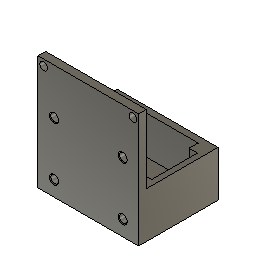
DigitalRegulator_mount_base v4 (Autodesk Fusion 360 design; units mm, degrees)
Autodesk Fusion 360 part; units mm, degrees
sketch "Sketch1" plane through (0, 0, 0) normal (0, 0, 1) x (1, 0, 0)
  line L0 (0, 0) -> (60, 0)
  line L1 (60, 0) -> (60, 50)
  line L2 (60, 50) -> (0, 50)
  line L3 (0, 50) -> (0, 0)
  dimension "d1" = 60
  dimension "d2" = 50
  constraint horizontal L0
  constraint vertical L1
  constraint horizontal L2
  constraint vertical L3
  constraint coincident L0.start L3.end
  measures "d1" distance of L0.start L0.end
  measures "d2" distance of L0.start L2.end
extrude "Extrude1" add sketch "Sketch1" along normal blind 30
sketch "Sketch2" plane through (0, 0, 30) normal (0, 0, 1) x (-1, 0, 0)
  line L0 (0, -50) -> (0, 0)
  line L1 (0, 0) -> (-60, 0)
  line L2 (-60, 0) -> (-60, -50)
  line L3 (-60, -50) -> (0, -50)
  line L4 (-54, -5) -> (-6, -5)
  line L5 (-6, -5) -> (-6, -45)
  line L6 (-6, -45) -> (-54, -45)
  line L7 (-54, -45) -> (-54, -5)
  line L8 (-54, -5) -> (-6, -45) construction
  line L9 (-6, -5) -> (-54, -45) construction
  point P0 (-30, -25)
  dimension "d5" = 48
  dimension "d6" = 40
  constraint horizontal L4
  constraint perpendicular L4 L5
  constraint parallel L4 L6
  constraint parallel L5 L7
  constraint coincident L8 P0
  constraint coincident L9 P0
  measures "d5" distance of L5.end L6.end
  measures "d6" distance of L4.end L5.end
extrude "Extrude2" cut sketch "Sketch2" against normal blind 25 contours L4 L5 L6 L7
sketch "Sketch3" plane through (0, 0, 30) normal (0, 0, 1) x (-1, 0, 0)
  line L0 (-6, -5) -> (-6, -45)
  line L1 (-6, -45) -> (-54, -45)
  line L2 (-54, -45) -> (-54, -5)
  line L3 (-54, -5) -> (-6, -5)
  line L4 (0, -50) -> (0, 0)
  line L5 (0, 0) -> (-60, 0)
  line L6 (-60, 0) -> (-60, -50)
  line L7 (-60, -50) -> (0, -50)
  line L8 (-54, -10) -> (-59.5, -10)
  line L9 (-59.5, -10) -> (-59.5, -40)
  line L10 (-59.5, -40) -> (-54, -40)
  line L11 (-54, -40) -> (-54, -10)
  line L12 (-6, -10) -> (-0.5, -10)
  line L13 (-0.5, -10) -> (-0.5, -40)
  line L14 (-0.5, -40) -> (-6, -40)
  line L15 (-6, -40) -> (-6, -10)
  dimension "d9" = 5.5
  dimension "d10" = 30
  dimension "d11" = 5.5
  dimension "d12" = 30
  constraint horizontal L8
  constraint vertical L9
  constraint horizontal L10
  constraint vertical L11
  constraint coincident L2 L8.start
  constraint horizontal L12
  constraint vertical L13
  constraint horizontal L14
  constraint vertical L15
  constraint coincident L0 L12.start
  measures "d9" distance of L8.start L8.end
  measures "d10" distance of L8.start L10.end
  measures "d11" distance of L12.start L12.end
  measures "d12" distance of L12.start L14.end
extrude "Extrude3" cut sketch "Sketch3" against normal blind 10 contours L0 L12 L13 L14 L15 | L2 L8 L9 L10 L11
move_face "OffsetFaces1" offset 3 1 faces at (0, 33.3333, 10)
move_face "OffsetFaces2" offset 3 1 faces at (60, 33.3333, 20)
move_face "OffsetFaces3" offset 2 1 faces at (19, 0, 20)
sketch "Sketch4" plane through (0, 0, 30) normal (0, 0, 1) x (-1, 0, 0)
  line L0 (-59.5, -10) -> (-54, -10)
  line L1 (-54, -10) -> (-54, -5)
  line L2 (-54, -5) -> (-6, -5)
  line L3 (-6, -5) -> (-6, -10)
  line L4 (-6, -10) -> (-0.5, -10)
  line L5 (-0.5, -10) -> (-0.5, -40)
  line L6 (-0.5, -40) -> (-6, -40)
  line L7 (-6, -40) -> (-6, -45)
  line L8 (-6, -45) -> (-54, -45)
  line L9 (-54, -45) -> (-54, -40)
  line L10 (-54, -40) -> (-59.5, -40)
  line L11 (-59.5, -40) -> (-59.5, -10)
  line L12 (3, -50) -> (3, 2)
  line L13 (3, 2) -> (-63, 2)
  line L14 (-63, 2) -> (-63, -50)
  line L15 (-63, -50) -> (3, -50)
  line L16 (3, 2) -> (-63, 2)
  line L17 (-63, 2) -> (-63, -3)
  line L18 (-63, -3) -> (3, -3)
  line L19 (3, -3) -> (3, 2)
  dimension "d18" = 66
  dimension "d19" = 5
  constraint horizontal L16
  constraint vertical L17
  constraint horizontal L18
  constraint vertical L19
  constraint coincident L12.end L13.start
  measures "d18" distance of L12.end L13.end
  measures "d19" distance of L12.end L18.end
extrude "Extrude4" add sketch "Sketch4" along normal blind 45 contours L12 L13 L14 L16 L17 L18 L19
sketch "Sketch7" plane through (0, 3, 0) normal (0, 1, 0) x (-1, 0, 0)
  line L0 (-63, 30) -> (3, 30)
  line L1 (3, 30) -> (3, 75)
  line L2 (3, 75) -> (-63, 75)
  line L3 (-63, 75) -> (-63, 30)
  point P0 (-59.25, 71)
  point P1 (-0.75, 71)
hole "Hole1" at (59.25, 3, 71) at (0.75, 3, 71) direction (0, -1, 0) diameter 5.1 depth 130 tip angle 118 countersink diameter 6 countersink angle 90
sketch "Sketch8" plane through (0, -2, 0) normal (0, -1, 0) x (1, 0, 0)
  circle A0 centre (59.25, 71) radius 2.55
  circle A1 centre (0.75, 71) radius 2.55
  line L0 (-3, 0) -> (63, 0)
  line L1 (63, 0) -> (63, 75)
  line L2 (63, 75) -> (-3, 75)
  line L3 (-3, 75) -> (-3, 0)
  point P0 (52.5, 45)
  point P1 (7.5, 45)
  constraint horizontal P0 P1
hole "Hole2" at (7.5, -2, 45) at (52.5, -2, 45) direction (0, 1, 0) diameter 5.1 depth 130 tip angle 118 countersink diameter 6 countersink angle 90
sketch "Sketch9" plane through (0, -2, 0) normal (0, -1, 0) x (1, 0, 0)
  circle A0 centre (7.5, 45) radius 3
  circle A1 centre (52.5, 45) radius 3
  circle A2 centre (59.25, 71) radius 2.55
  circle A3 centre (0.75, 71) radius 2.55
  line L0 (-3, 0) -> (63, 0)
  line L1 (63, 0) -> (63, 75)
  line L2 (63, 75) -> (-3, 75)
  line L3 (-3, 75) -> (-3, 0)
  point P0 (7.5, 10)
  point P1 (52.5, 10)
  constraint horizontal P0 P1
hole "Hole3" at (7.5, -2, 10) at (52.5, -2, 10) direction (0, 1, 0) diameter 5.1 depth 5.6 tip angle 180 countersink diameter 6 countersink angle 90
sketch "Sketch10" plane through (6, 0, 0) normal (1, 0, 0) x (0, 1, 0)
  line L0 (40, 30) -> (40, 20)
  line L1 (40, 20) -> (10, 20)
  line L2 (10, 20) -> (10, 30)
  line L3 (10, 30) -> (5, 30)
  line L4 (5, 30) -> (5, 5)
  line L5 (5, 5) -> (45, 5)
  line L6 (45, 5) -> (45, 30)
  line L7 (45, 30) -> (40, 30)
  line L8 (23.25, 30) -> (26.75, 30)
  line L9 (26.75, 30) -> (26.75, 0)
  line L10 (26.75, 0) -> (23.25, 0)
  line L11 (23.25, 0) -> (23.25, 30)
  point P0 (23.25, 30)
  dimension "d41" = 3.5
  constraint horizontal L8
  constraint vertical L9
  constraint horizontal L10
  constraint vertical L11
  constraint coincident P0 L8.start
  measures "d41" distance of P0 L8.end
extrude "Extrude5" cut sketch "Sketch10" against normal blind 1 contours L1 L5 L9 L11
sketch "Sketch11" plane through (54, 0, 0) normal (-1, 0, 0) x (0, -1, 0)
  line L0 (-10, 30) -> (-10, 20)
  line L1 (-10, 20) -> (-40, 20)
  line L2 (-40, 20) -> (-40, 30)
  line L3 (-40, 30) -> (-45, 30)
  line L4 (-45, 30) -> (-45, 5)
  line L5 (-45, 5) -> (-5, 5)
  line L6 (-5, 5) -> (-5, 30)
  line L7 (-5, 30) -> (-10, 30)
  line L8 (-23.25, 30) -> (-26.75, 30)
  line L9 (-26.75, 30) -> (-26.75, 0)
  line L10 (-26.75, 0) -> (-23.25, 0)
  line L11 (-23.25, 0) -> (-23.25, 30)
  point P0 (-23.25, 30)
  dimension "d44" = 3.5
  constraint horizontal L8
  constraint vertical L9
  constraint horizontal L10
  constraint vertical L11
  constraint coincident P0 L8.start
  measures "d44" distance of P0 L8.end
extrude "Extrude6" cut sketch "Sketch11" against normal blind 1 contours L1 L5 L9 L11
move_face "OffsetFaces4" offset -1 1 faces at (22, 45, 21.6667)
move_face "OffsetFaces5" offset -0.5 1 faces at (38, 5, 13.3333)
